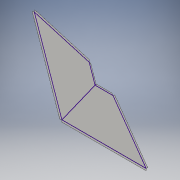
# Autodesk Inventor part: DELL screen 3D hologram piece
Saved by Autodesk Inventor 2016 (Build 200138000, 138)
## iProperties
Created: 2017-09-08
Part Number: DELL screen 3D hologram piece
Material: Generic
Document SubType Name: Modeling
Designer: student
Density: 1 g/cm^3
Appearance: Default
Author: student
Autodesk Inventor part; units mm, degrees
ref_plane "YZ Plane" through (0, 0, 0) normal (1, 0, 0) x (0, 1, 0)
ref_plane "XZ Plane" through (0, 0, 0) normal (0, 1, 0) x (-1, 0, 0)
ref_plane "XY Plane" through (0, 0, 0) normal (0, 0, 1) x (1, 0, 0)
sketch "Sketch1" plane through (0, 0, 0) normal (0, 0, 1) x (1, 0, 0)
  line L0 (-149.2247, -82.55) -> (149.2253, -82.55)
  line L1 (31.75, 82.55) -> (-31.75, 82.55)
  line L2 (31.75, 82.55) -> (149.2253, -82.55)
  line L3 (-31.75, 82.55) -> (-149.2247, -82.55)
  line L4 (-149.2247, -82.55) -> (-247.0638, 199.4073)
  line L5 (-31.75, 82.55) -> (-52.5668, 142.5409)
  line L6 (-247.0638, 199.4073) -> (-52.5668, 142.5409)
  point P0 (0, 0)
  point P1 (0, 82.55)
  point P2 (-90.4873, 0)
  dimension "d1" = 298.45
  dimension "d2" = 63.5
  dimension "d3" = 165.1
  dimension "d4" = 202.6285
  dimension "d5" = 202.6289
  dimension "d31" = 125.433
  dimension "d32" = 125.433
  dimension "d33" = 54.567
  dimension "d34" = 54.567
  dimension "d35" = 54.57
  dimension "d36" = 298.45
  dimension "d37" = 125.43
  dimension "d38" = 63.5
  dimension "d39" = 202.6397
  dimension "d40" = 54.566
  dimension "d41" = 125.434
  constraints: 14 end point, 2 midpoint, 1 horizontal, 1 horizontal alignment, 1 parallel, 1 vertical alignment
  measures "d1" distance of L0.start L0.end
  measures "d2" distance of L1.start L1.end
  measures "d3" distance between parallel lines of L0 L1
  measures "d4" distance of L1.end L0.start
  measures "d5" distance of L1.start L0.end
  measures "d31" angle of L3 L1
  measures "d32" angle of L2 L1
  measures "d33" angle of L0 L2
  measures "d34" angle of L0 L3
  measures "d35" angle of L4 L3
  measures "d36" distance of L0.start L4.end
  measures "d37" angle of L3 L5
  measures "d38" distance of L1.end L5.end
  measures "d39" distance of L4.end L5.end
  measures "d40" angle of L4 L6
  measures "d41" angle of L5 L6
extrude "Extrusion2" add sketch "Sketch1" along normal blind 0.127
sketch "Sketch3" plane through (0, 0, 0.127) normal (0, 0, 1) x (1, 0, 0)
  line L0 (31.75, 82.55) -> (-31.75, 82.55) projected
  line L1 (-31.75, 82.55) -> (31.75, 82.55)
  line L2 (-31.75, 82.55) -> (-28.1358, 87.63)
  line L3 (31.75, 82.55) -> (28.1358, 87.63)
  line L4 (-28.1358, 87.63) -> (28.1358, 87.63)
  line L5 (-31.75, 82.55) -> (-52.5668, 142.5409) projected
  line L6 (-52.5668, 142.5409) -> (-46.5827, 140.7918)
  line L7 (-46.5827, 140.7918) -> (-28.1358, 87.63)
  line L8 (-149.2247, -82.55) -> (149.2253, -82.55) projected
  line L9 (-52.5668, 142.5409) -> (-247.0638, 199.4073) projected
  line L10 (-247.0638, 199.4073) -> (-149.2247, -82.55) projected
  line L11 (149.2253, -82.55) -> (149.2253, -90.17)
  line L12 (149.2253, -90.17) -> (-149.2247, -90.17)
  line L13 (-149.2247, -90.17) -> (-149.2247, -82.55)
  line L14 (-247.0638, 199.4073) -> (-149.2247, -82.55) projected
  line L15 (-149.2247, -82.55) -> (-156.4236, -85.048)
  line L16 (-156.4236, -85.048) -> (-254.2627, 196.9093)
  line L17 (-254.2627, 196.9093) -> (-247.0638, 199.4073)
  line L18 (-247.0638, 199.4073) -> (-244.9254, 206.7211)
  line L19 (-244.9254, 206.7211) -> (-50.4284, 149.8547)
  line L20 (-50.4284, 149.8547) -> (-52.5668, 142.5409)
  line L21 (-31.75, 82.55) -> (31.75, 82.55)
  line L22 (149.2253, -82.55) -> (31.75, 82.55) projected
  line L23 (31.75, 82.55) -> (37.9587, 86.9677)
  line L24 (37.9587, 86.9677) -> (155.434, -78.1323)
  line L25 (149.2253, -82.55) -> (155.434, -78.1323)
  line L26 (31.75, 82.55) -> (149.2253, -82.55)
  line L27 (-52.5668, 142.5409) -> (-31.75, 82.55)
  line L28 (-46.5827, 140.7918) -> (-28.1358, 87.63)
  line L29 (-28.1358, 87.63) -> (28.1358, 87.63)
  point P0 (0, 0)
  dimension "d45" = 54.57
  dimension "d46" = 5.08
  dimension "d47" = 54.57
  dimension "d48" = 54.57
  dimension "d51" = 5.08
  dimension "d66" = 7.62
  dimension "d67" = 90
  dimension "d68" = 7.62
  dimension "d72" = 90
  dimension "d73" = 7.62
  dimension "d76" = 7.62
  dimension "d77" = 90
  dimension "d80" = 90
  dimension "d81" = 7.62
  dimension "d82" = 90
  dimension "d83" = 7.62
  dimension "d84" = 7.62
  dimension "d85" = 7.62
  constraints: 46 end point, 6 perpendicular, 3 horizontal, 2 parallel, 1 collinear, 1 vertical
  measures "d45" angle of L0 L2
  measures "d46" distance from line of L2.end L0
  measures "d47" angle of L0 L3
  measures "d48" angle of L5 L6
  measures "d51" distance from line of L5 L6.end
  measures "d66" distance of L8.end L11.end
  measures "d67" angle of L14 L15
  measures "d68" distance from line of L10 L16.end
  measures "d72" angle of L9 L18
  measures "d73" distance from line of L9 L18.end
  measures "d76" distance from line of L9 L19.end
  measures "d77" angle of L9 L20
  measures "d80" angle of L22 L23
  measures "d81" distance from line of L22 L23.end
  measures "d82" angle of L22 L25
  measures "d83" distance from line of L22 L24.end
  measures "d84" distance from line of L10 L15.end
  measures "d85" distance from line of L8 L12.end
extrude "Extrusion4" add sketch "Sketch3" along normal blind 0.127
sketch "Sketch5" plane through (0, 0, 0.254) normal (0, 0, 1) x (1, 0, 0)
  line L0 (31.75, 82.55) -> (-31.75, 82.55) projected
  line L1 (31.75, 82.55) -> (-31.75, 82.55)
  line L2 (-149.2247, -82.55) -> (149.2253, -82.55) projected
  line L3 (31.75, 82.55) -> (149.2253, -82.55)
  line L4 (149.2253, -82.55) -> (-149.2247, -82.55)
  line L5 (-247.0638, 199.4073) -> (-149.2247, -82.55) projected
  line L6 (-149.2247, -82.55) -> (-247.0638, 199.4073)
  line L7 (-247.0638, 199.4073) -> (-52.5668, 142.5409)
  line L8 (-31.75, 82.55) -> (-52.5668, 142.5409) projected
  line L9 (-52.5668, 142.5409) -> (-31.75, 82.55)
  line L10 (-31.75, 82.55) -> (-28.1358, 87.63)
  line L11 (-31.75, 82.55) -> (-149.2247, -82.55)
  constraints: 16 end point, 3 collinear, 1 horizontal
body "Solid2"
